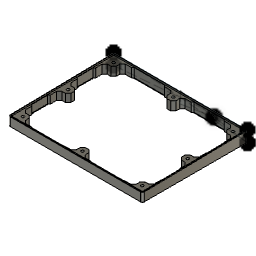
case (Autodesk Fusion 360 design; units mm, degrees)
Autodesk Fusion 360 part; units mm, degrees
sketch "Sketch1" plane through (0, 0, 0) normal (0, 0, 1) x (1, 0, 0)
  line L0 (0, 0) -> (294.692, 0)
  line L1 (294.692, 0) -> (294.692, 230.4)
  line L2 (294.692, 230.4) -> (0, 230.4)
  line L3 (0, 230.4) -> (0, 0)
  line L4 (-2, 232.4) -> (296.692, 232.4)
  line L5 (296.692, 232.4) -> (296.692, -2)
  line L6 (296.692, -2) -> (-2, -2)
  line L7 (-2, -2) -> (-2, 232.4)
  line L8 (4, 226.4) -> (290.692, 226.4)
  line L9 (290.692, 226.4) -> (290.692, 4)
  line L10 (290.692, 4) -> (4, 4)
  line L11 (4, 4) -> (4, 226.4)
  line L12 (-2, 232.4) -> (296.692, -2) construction
  line L13 (-2, -2) -> (296.692, 232.4) construction
  line L14 (147.346, 232.4) -> (147.346, -2) construction
  line L15 (296.692, 115.2) -> (-2, 115.2) construction
  line L16 (4, 226.4) -> (24, 226.4)
  line L17 (24, 226.4) -> (24, 206.4)
  line L18 (24, 206.4) -> (4, 206.4)
  line L19 (4, 206.4) -> (4, 226.4)
  line L20 (137.346, 226.4) -> (157.346, 226.4)
  line L21 (157.346, 226.4) -> (157.346, 206.4)
  line L22 (157.346, 206.4) -> (137.346, 206.4)
  line L23 (137.346, 206.4) -> (137.346, 226.4)
  line L24 (290.692, 226.4) -> (270.692, 226.4)
  line L25 (270.692, 226.4) -> (270.692, 206.4)
  line L26 (270.692, 206.4) -> (290.692, 206.4)
  line L27 (290.692, 206.4) -> (290.692, 226.4)
  line L28 (4, 125.2) -> (24, 125.2)
  line L29 (24, 125.2) -> (24, 105.2)
  line L30 (24, 105.2) -> (4, 105.2)
  line L31 (4, 105.2) -> (4, 125.2)
  line L32 (290.692, 125.2) -> (270.692, 125.2)
  line L33 (270.692, 125.2) -> (270.692, 105.2)
  line L34 (270.692, 105.2) -> (290.692, 105.2)
  line L35 (290.692, 105.2) -> (290.692, 125.2)
  line L36 (4, 4) -> (24, 4)
  line L37 (24, 4) -> (24, 24)
  line L38 (24, 24) -> (4, 24)
  line L39 (4, 24) -> (4, 4)
  line L40 (137.346, 4) -> (157.346, 4)
  line L41 (157.346, 4) -> (157.346, 24)
  line L42 (157.346, 24) -> (137.346, 24)
  line L43 (137.346, 24) -> (137.346, 4)
  line L44 (290.692, 4) -> (270.692, 4)
  line L45 (270.692, 4) -> (270.692, 24)
  line L46 (270.692, 24) -> (290.692, 24)
  line L47 (290.692, 24) -> (290.692, 4)
  line L48 (4, 206.4) -> (24, 226.4) construction
  line L49 (4, 226.4) -> (24, 206.4) construction
  line L50 (137.346, 226.4) -> (157.346, 206.4) construction
  line L51 (137.346, 206.4) -> (157.346, 226.4) construction
  line L52 (270.692, 226.4) -> (290.692, 206.4) construction
  line L53 (270.692, 206.4) -> (290.692, 226.4) construction
  line L54 (290.692, 125.2) -> (270.692, 105.2) construction
  line L55 (270.692, 125.2) -> (290.692, 105.2) construction
  line L56 (270.692, 4) -> (290.692, 24) construction
  line L57 (270.692, 24) -> (290.692, 4) construction
  line L58 (137.346, 4) -> (157.346, 24) construction
  line L59 (137.346, 24) -> (157.346, 4) construction
  line L60 (24, 24) -> (4, 4) construction
  line L61 (4, 24) -> (24, 4) construction
  line L62 (4, 125.2) -> (24, 105.2) construction
  line L63 (4, 105.2) -> (24, 125.2) construction
  circle A0 centre (14, 216.4) radius 3
  circle A1 centre (147.346, 216.4) radius 3
  circle A2 centre (14, 115.2) radius 3
  circle A3 centre (14, 14) radius 3
  circle A4 centre (147.346, 14) radius 3
  circle A5 centre (280.692, 14) radius 3
  circle A6 centre (280.692, 115.2) radius 3
  circle A7 centre (280.692, 216.4) radius 3
  line L64 (44, 226.4) -> (44, 230.4)
  line L65 (117.346, 230.4) -> (177.346, 230.4)
  line L66 (177.346, 230.4) -> (177.346, 226.4)
  line L67 (177.346, 226.4) -> (117.346, 226.4)
  line L68 (117.346, 226.4) -> (117.346, 230.4)
  line L69 (250.692, 226.4) -> (250.692, 230.4)
  line L70 (290.692, 186.4) -> (294.692, 186.4)
  line L71 (4, 186.4) -> (0, 186.4)
  line L72 (0, 145.2) -> (4, 145.2)
  line L73 (4, 145.2) -> (4, 85.2)
  line L74 (4, 85.2) -> (0, 85.2)
  line L75 (0, 85.2) -> (0, 145.2)
  line L76 (294.692, 145.2) -> (290.692, 145.2)
  line L77 (290.692, 145.2) -> (290.692, 85.2)
  line L78 (290.692, 85.2) -> (294.692, 85.2)
  line L79 (294.692, 85.2) -> (294.692, 145.2)
  line L80 (4, 44) -> (0, 44)
  line L81 (44, 4) -> (44, 0)
  line L82 (117.346, 4) -> (177.346, 4)
  line L83 (177.346, 4) -> (177.346, 0)
  line L84 (177.346, 0) -> (117.346, 0)
  line L85 (117.346, 0) -> (117.346, 4)
  line L86 (250.692, 4) -> (250.692, 0)
  line L87 (290.692, 44) -> (294.692, 44)
  line L88 (250.692, 1) -> (177.346, 1)
  line L89 (250.692, 4) -> (246.692, 0)
  line L90 (177.346, 4) -> (181.346, 0)
  line L91 (293.692, 44) -> (293.692, 85.2)
  line L92 (290.692, 44) -> (294.692, 48)
  line L93 (290.692, 85.2) -> (294.692, 81.2)
  line L94 (250.692, 229.4) -> (177.346, 229.4)
  line L95 (250.692, 226.4) -> (246.692, 230.4)
  line L96 (177.346, 226.4) -> (181.346, 230.4)
  line L97 (117.346, 1) -> (44, 1)
  line L98 (117.346, 4) -> (113.346, 0)
  line L99 (44, 4) -> (48, 0)
  line L100 (1, 44) -> (1, 85.2)
  line L101 (4, 44) -> (0, 48)
  line L102 (4, 85.2) -> (0, 81.2)
  line L103 (1, 186.4) -> (1, 145.2)
  line L104 (4, 186.4) -> (0, 182.4)
  line L105 (4, 145.2) -> (0, 149.2)
  line L106 (117.346, 229.4) -> (44, 229.4)
  line L107 (117.346, 226.4) -> (113.346, 230.4)
  line L108 (44, 226.4) -> (48, 230.4)
  line L109 (293.692, 145.2) -> (293.692, 186.4)
  line L110 (290.692, 145.2) -> (294.692, 149.2)
  line L111 (290.692, 186.4) -> (294.692, 182.4)
  dimension "d1" = 294.692
  dimension "d2" = 230.4
  dimension "d3" = 2
  dimension "d4" = 2
  dimension "d5" = 2
  dimension "d6" = 2
  dimension "d7" = 4
  dimension "d8" = 4
  dimension "d9" = 4
  dimension "d10" = 4
  dimension "d11" = 20
  dimension "d12" = 20
  dimension "d13" = 20
  dimension "d14" = 20
  dimension "d15" = 20
  dimension "d16" = 20
  dimension "d17" = 20
  dimension "d18" = 20
  dimension "d19" = 20
  dimension "d20" = 20
  dimension "d21" = 20
  dimension "d22" = 20
  dimension "d23" = 20
  dimension "d24" = 20
  dimension "d25" = 20
  dimension "d26" = 20
  dimension "d27" = 6
  dimension "d28" = 6
  dimension "d29" = 6
  dimension "d30" = 6
  dimension "d31" = 6
  dimension "d32" = 6
  dimension "d33" = 6
  dimension "d34" = 6
  dimension "d35" = 20
  dimension "d36" = 20
  dimension "d37" = 20
  dimension "d38" = 20
  dimension "d39" = 20
  dimension "d40" = 20
  dimension "d41" = 20
  dimension "d42" = 20
  dimension "d43" = 20
  dimension "d44" = 20
  dimension "d45" = 20
  dimension "d46" = 20
  dimension "d47" = 20
  dimension "d48" = 20
  dimension "d49" = 20
  dimension "d50" = 20
  dimension "d51" = 1
  dimension "d52" = 4
  dimension "d53" = 4
  dimension "d54" = 1
  dimension "d55" = 4
  dimension "d56" = 4
  dimension "d57" = 1
  dimension "d58" = 4
  dimension "d59" = 4
  dimension "d60" = 1
  dimension "d61" = 4
  dimension "d62" = 4
  dimension "d63" = 1
  dimension "d64" = 4
  dimension "d65" = 4
  dimension "d66" = 1
  dimension "d67" = 4
  dimension "d68" = 4
  dimension "d69" = 1
  dimension "d70" = 4
  dimension "d71" = 4
  dimension "d72" = 1
  dimension "d73" = 4
  dimension "d74" = 4
  constraint horizontal L0
  constraint vertical L1
  constraint horizontal L2
  constraint vertical L3
  constraint coincident L0.start L3.end
  constraint horizontal L4
  constraint vertical L5
  constraint horizontal L6
  constraint vertical L7
  constraint horizontal L8
  constraint vertical L9
  constraint horizontal L10
  constraint vertical L11
  constraint midpoint L4 L14.start
  constraint midpoint L6 L14.end
  constraint midpoint L5 L15.start
  constraint midpoint L7 L15.end
  constraint horizontal L16
  constraint vertical L17
  constraint horizontal L18
  constraint vertical L19
  constraint horizontal L20
  constraint vertical L21
  constraint horizontal L22
  constraint vertical L23
  constraint coincident L8 L20.start
  constraint horizontal L24
  constraint vertical L25
  constraint horizontal L26
  constraint vertical L27
  constraint horizontal L28
  constraint vertical L29
  constraint horizontal L30
  constraint vertical L31
  constraint coincident L11 L28.start
  constraint horizontal L32
  constraint vertical L33
  constraint horizontal L34
  constraint vertical L35
  constraint coincident L9 L32.start
  constraint horizontal L36
  constraint vertical L37
  constraint horizontal L38
  constraint vertical L39
  constraint horizontal L40
  constraint vertical L41
  constraint horizontal L42
  constraint vertical L43
  constraint coincident L10 L40.start
  constraint horizontal L44
  constraint vertical L45
  constraint horizontal L46
  constraint vertical L47
  constraint symmetric L14 L21 L23
  constraint symmetric L15 L28 L30
  constraint symmetric L15 L32 L34
  constraint symmetric L14 L41 L43
  constraint midpoint L48 A0.centre
  constraint midpoint L50 A1.centre
  constraint midpoint L63 A2.centre
  constraint midpoint L61 A3.centre
  constraint midpoint L59 A4.centre
  constraint midpoint L57 A5.centre
  constraint midpoint L55 A6.centre
  constraint midpoint L52 A7.centre
  constraint coincident L8 L64.start
  constraint coincident L2 L64.end
  constraint perpendicular L2 L64
  constraint horizontal L65
  constraint vertical L66
  constraint horizontal L67
  constraint vertical L68
  constraint coincident L8 L66.end
  constraint coincident L2 L65.start
  constraint coincident L8 L69.start
  constraint coincident L2 L69.end
  constraint perpendicular L2 L69
  constraint coincident L9 L70.start
  constraint coincident L1 L70.end
  constraint perpendicular L1 L70
  constraint coincident L11 L71.start
  constraint coincident L3 L71.end
  constraint perpendicular L3 L71
  constraint horizontal L72
  constraint vertical L73
  constraint horizontal L74
  constraint vertical L75
  constraint coincident L11 L73.end
  constraint coincident L3 L72.start
  constraint horizontal L76
  constraint vertical L77
  constraint horizontal L78
  constraint vertical L79
  constraint coincident L9 L77.end
  constraint coincident L1 L76.start
  constraint coincident L11 L80.start
  constraint coincident L3 L80.end
  constraint perpendicular L3 L80
  constraint coincident L10 L81.start
  constraint coincident L0 L81.end
  constraint perpendicular L0 L81
  constraint horizontal L82
  constraint vertical L83
  constraint horizontal L84
  constraint vertical L85
  constraint coincident L0 L83.end
  constraint coincident L10 L82.start
  constraint coincident L10 L86.start
  constraint coincident L0 L86.end
  constraint perpendicular L0 L86
  constraint coincident L9 L87.start
  constraint coincident L1 L87.end
  constraint perpendicular L1 L87
  constraint coincident L86 L88.start
  constraint coincident L83 L88.end
  constraint perpendicular L83 L88
  constraint coincident L0 L89.end
  constraint coincident L0 L90.end
  constraint coincident L87 L91.start
  constraint coincident L78 L91.end
  constraint perpendicular L78 L91
  constraint coincident L1 L92.end
  constraint coincident L1 L93.end
  constraint coincident L69 L94.start
  constraint coincident L66 L94.end
  constraint perpendicular L66 L94
  constraint coincident L2 L95.end
  constraint coincident L2 L96.end
  constraint coincident L85 L97.start
  constraint coincident L81 L97.end
  constraint perpendicular L81 L97
  constraint coincident L0 L98.end
  constraint coincident L0 L99.end
  constraint coincident L80 L100.start
  constraint coincident L74 L100.end
  constraint perpendicular L74 L100
  constraint coincident L3 L101.end
  constraint coincident L3 L102.end
  constraint coincident L71 L103.start
  constraint coincident L72 L103.end
  constraint perpendicular L72 L103
  constraint coincident L3 L104.end
  constraint coincident L3 L105.end
  constraint coincident L68 L106.start
  constraint coincident L64 L106.end
  constraint perpendicular L64 L106
  constraint coincident L2 L107.end
  constraint coincident L2 L108.end
  constraint coincident L76 L109.start
  constraint coincident L70 L109.end
  constraint perpendicular L70 L109
  constraint coincident L1 L110.end
  constraint coincident L1 L111.end
  measures "d1" distance of L0.start L0.end
  measures "d2" distance of L0.start L2.end
  measures "d3" distance of L3 L7
  measures "d4" distance of L2 L4
  measures "d5" distance of L1 L5
  measures "d6" distance of L0 L6
  measures "d7" distance of L2 L8
  measures "d8" distance of L3 L11
  measures "d9" distance of L1 L9
  measures "d10" distance of L0 L10
  measures "d11" distance of L8.start L16.end
  measures "d12" distance of L8.start L18.end
  measures "d13" distance of L20.start L20.end
  measures "d14" distance of L20.start L22.end
  measures "d15" distance of L8.end L24.end
  measures "d16" distance of L8.end L26.end
  measures "d17" distance of L28.start L28.end
  measures "d18" distance of L28.start L30.end
  measures "d19" distance of L32.start L32.end
  measures "d20" distance of L32.start L34.end
  measures "d21" distance of L10.end L36.end
  measures "d22" distance of L10.end L38.end
  measures "d23" distance of L40.start L40.end
  measures "d24" distance of L40.start L42.end
  measures "d25" distance of L9.end L44.end
  measures "d26" distance of L9.end L46.end
  measures "d27" diameter of A0
  measures "d28" diameter of A1
  measures "d29" diameter of A2
  measures "d30" diameter of A3
  measures "d31" diameter of A4
  measures "d32" diameter of A5
  measures "d33" diameter of A6
  measures "d34" diameter of A7
  measures "d35" distance of L16.end L64.start
  measures "d36" distance of L20.start L67.end
  measures "d37" distance of L20.end L66.end
  measures "d38" distance of L24.end L69.start
  measures "d39" distance of L26.end L70.start
  measures "d40" distance of L18.end L71.start
  measures "d41" distance of L28.start L72.end
  measures "d42" distance of L30.end L73.end
  measures "d43" distance of L32.start L76.end
  measures "d44" distance of L34.end L77.end
  measures "d45" distance of L38.end L80.start
  measures "d46" distance of L36.end L81.start
  measures "d47" distance of L40.start L82.start
  measures "d48" distance of L40.end L82.end
  measures "d49" distance of L44.end L86.start
  measures "d50" distance of L46.end L87.start
  measures "d51" distance of L0 L88
  measures "d52" distance of L86.end L89.end
  measures "d53" distance of L83.end L90.end
  measures "d54" distance of L1 L91
  measures "d55" distance of L87.end L92.end
  measures "d56" distance of L78.end L93.end
  measures "d57" distance of L2 L94
  measures "d58" distance of L69.end L95.end
  measures "d59" distance of L65.end L96.end
  measures "d60" distance of L0 L97
  measures "d61" distance of L84.end L98.end
  measures "d62" distance of L81.end L99.end
  measures "d63" distance of L3 L100
  measures "d64" distance of L80.end L101.end
  measures "d65" distance of L74.end L102.end
  measures "d66" distance of L3 L103
  measures "d67" distance of L71.end L104.end
  measures "d68" distance of L72.start L105.end
  measures "d69" distance of L2 L106
  measures "d70" distance of L65.start L107.end
  measures "d71" distance of L64.end L108.end
  measures "d72" distance of L1 L109
  measures "d73" distance of L76.start L110.end
  measures "d74" distance of L70.end L111.end
extrude "Extrude1" add sketch "Sketch1" along normal blind 20 contours L0 L3 L10 L11 L36 L39 L80 L81 | L0 L81 L97 L99 | L3 L80 L100 L101 | L0 L97 L98 L99 | L81 L97 L99 | L3 L100 L101 L102 | L80 L100 L101 | L0 L85 L97 L98 | L3 L74 L100 L102 | L0 L10 L40 L82 L83 L84 L85 | L85 L97 L98 | L10 L11 L36 L37 L38 L39 | L3 L11 L31 L72 L73 L74 L75 | L74 L100 L102 | L0 L83 L88 L90 | L10 L40 L41 L42 L43 L82 | L3 L72 L103 L105 | L11 L28 L29 L30 L31 L73 | L0 L88 L89 L90 | L83 L88 L90 | L3 L103 L104 L105 | L72 L103 L105 | L0 L86 L88 L89 | L3 L71 L103 L104 | L0 L1 L9 L10 L44 L47 L86 L87 | L86 L88 L89 | L2 L3 L8 L11 L16 L19 L64 L71 | L71 L103 L104 | L9 L10 L44 L45 L46 L47 | L8 L11 L16 L17 L18 L19 | L1 L87 L91 L92 | L2 L64 L106 L108 | L1 L91 L92 L93 | L87 L91 L92 | L2 L106 L107 L108 | L64 L106 L108 | L1 L78 L91 L93 | L2 L68 L106 L107 | L1 L9 L35 L76 L77 L78 L79 | L78 L91 L93 | L2 L8 L20 L65 L66 L67 L68 | L68 L106 L107 | L1 L76 L109 L110 | L9 L32 L33 L34 L35 L77 | L2 L66 L94 L96 | L8 L20 L21 L22 L23 L67 | L1 L109 L110 L111 | L76 L109 L110 | L2 L94 L95 L96 | L66 L94 L96 | L1 L70 L109 L111 | L2 L69 L94 L95 | L1 L2 L8 L9 L24 L27 L69 L70 | L70 L109 L111 | L69 L94 L95 | L8 L9 L24 L25 L26 L27 | L4 L5 L6 L7
chamfer "Chamfer1" distance 6 angle 45 28 edges at (270.692, 4, 10) (270.692, 24, 10) (290.692, 24, 10) (290.692, 105.2, 10) (270.692, 105.2, 10) (270.692, 125.2, 10) (290.692, 125.2, 10) (157.346, 4, 10) (157.346, 24, 10) (137.346, 4, 10) (137.346, 24, 10) (290.692, 206.4, 10) (270.692, 206.4, 10) (270.692, 226.4, 10) (157.346, 206.4, 10) (157.346, 226.4, 10) (137.346, 206.4, 10) (137.346, 226.4, 10) (24, 206.4, 10) (24, 226.4, 10) (4, 206.4, 10) (4, 125.2, 10) (24, 125.2, 10) (24, 105.2, 10) (4, 105.2, 10) (4, 24, 10) (24, 24, 10) (24, 4, 10)
sketch "Sketch2" plane through (0, 0, 20) normal (0, 0, 1) x (-1, 0, 0)
  line L0 (-24, -18) -> (-18, -24)
  line L1 (-18, -24) -> (-10, -24)
  line L2 (-10, -24) -> (-4, -30)
  line L3 (-4, -30) -> (-4, -44)
  line L4 (-4, -44) -> (-1, -47)
  line L5 (-1, -47) -> (-1, -82.2)
  line L6 (-1, -82.2) -> (-4, -85.2)
  line L7 (-4, -85.2) -> (-4, -99.2)
  line L8 (-4, -99.2) -> (-10, -105.2)
  line L9 (-10, -105.2) -> (-18, -105.2)
  line L10 (-18, -105.2) -> (-24, -111.2)
  line L11 (-24, -111.2) -> (-24, -119.2)
  line L12 (-24, -119.2) -> (-18, -125.2)
  line L13 (-18, -125.2) -> (-10, -125.2)
  line L14 (-10, -125.2) -> (-4, -131.2)
  line L15 (-4, -131.2) -> (-4, -145.2)
  line L16 (-4, -145.2) -> (-1, -148.2)
  line L17 (-1, -148.2) -> (-1, -183.4)
  line L18 (-1, -183.4) -> (-4, -186.4)
  line L19 (-4, -186.4) -> (-4, -200.4)
  line L20 (-4, -200.4) -> (-10, -206.4)
  line L21 (-10, -206.4) -> (-18, -206.4)
  line L22 (-18, -206.4) -> (-24, -212.4)
  line L23 (-24, -212.4) -> (-24, -220.4)
  line L24 (-24, -220.4) -> (-30, -226.4)
  line L25 (-30, -226.4) -> (-44, -226.4)
  line L26 (-44, -226.4) -> (-47, -229.4)
  line L27 (-47, -229.4) -> (-114.346, -229.4)
  line L28 (-114.346, -229.4) -> (-117.346, -226.4)
  line L29 (-117.346, -226.4) -> (-131.346, -226.4)
  line L30 (-131.346, -226.4) -> (-137.346, -220.4)
  line L31 (-137.346, -220.4) -> (-137.346, -212.4)
  line L32 (-137.346, -212.4) -> (-143.346, -206.4)
  line L33 (-143.346, -206.4) -> (-151.346, -206.4)
  line L34 (-151.346, -206.4) -> (-157.346, -212.4)
  line L35 (-157.346, -212.4) -> (-157.346, -220.4)
  line L36 (-157.346, -220.4) -> (-163.346, -226.4)
  line L37 (-163.346, -226.4) -> (-177.346, -226.4)
  line L38 (-177.346, -226.4) -> (-180.346, -229.4)
  line L39 (-180.346, -229.4) -> (-247.692, -229.4)
  line L40 (-247.692, -229.4) -> (-250.692, -226.4)
  line L41 (-250.692, -226.4) -> (-264.692, -226.4)
  line L42 (-264.692, -226.4) -> (-270.692, -220.4)
  line L43 (-270.692, -220.4) -> (-270.692, -212.4)
  line L44 (-270.692, -212.4) -> (-276.692, -206.4)
  line L45 (-276.692, -206.4) -> (-284.692, -206.4)
  line L46 (-284.692, -206.4) -> (-290.692, -200.4)
  line L47 (-290.692, -200.4) -> (-290.692, -186.4)
  line L48 (-290.692, -186.4) -> (-293.692, -183.4)
  line L49 (-293.692, -183.4) -> (-293.692, -148.2)
  line L50 (-293.692, -148.2) -> (-290.692, -145.2)
  line L51 (-290.692, -145.2) -> (-290.692, -131.2)
  line L52 (-290.692, -131.2) -> (-284.692, -125.2)
  line L53 (-284.692, -125.2) -> (-276.692, -125.2)
  line L54 (-276.692, -125.2) -> (-270.692, -119.2)
  line L55 (-270.692, -119.2) -> (-270.692, -111.2)
  line L56 (-270.692, -111.2) -> (-276.692, -105.2)
  line L57 (-276.692, -105.2) -> (-284.692, -105.2)
  line L58 (-284.692, -105.2) -> (-290.692, -99.2)
  line L59 (-290.692, -99.2) -> (-290.692, -85.2)
  line L60 (-290.692, -85.2) -> (-293.692, -82.2)
  line L61 (-293.692, -82.2) -> (-293.692, -47)
  line L62 (-293.692, -47) -> (-290.692, -44)
  line L63 (-290.692, -44) -> (-290.692, -30)
  line L64 (-290.692, -30) -> (-284.692, -24)
  line L65 (-284.692, -24) -> (-276.692, -24)
  line L66 (-276.692, -24) -> (-270.692, -18)
  line L67 (-270.692, -18) -> (-270.692, -10)
  line L68 (-270.692, -10) -> (-264.692, -4)
  line L69 (-264.692, -4) -> (-250.692, -4)
  line L70 (-250.692, -4) -> (-247.692, -1)
  line L71 (-247.692, -1) -> (-180.346, -1)
  line L72 (-180.346, -1) -> (-177.346, -4)
  line L73 (-177.346, -4) -> (-163.346, -4)
  line L74 (-163.346, -4) -> (-157.346, -10)
  line L75 (-157.346, -10) -> (-157.346, -18)
  line L76 (-157.346, -18) -> (-151.346, -24)
  line L77 (-151.346, -24) -> (-143.346, -24)
  line L78 (-143.346, -24) -> (-137.346, -18)
  line L79 (-137.346, -18) -> (-137.346, -10)
  line L80 (-137.346, -10) -> (-131.346, -4)
  line L81 (-131.346, -4) -> (-117.346, -4)
  line L82 (-117.346, -4) -> (-114.346, -1)
  line L83 (-114.346, -1) -> (-47, -1)
  line L84 (-47, -1) -> (-44, -4)
  line L85 (-44, -4) -> (-30, -4)
  line L86 (-30, -4) -> (-24, -10)
  line L87 (-24, -10) -> (-24, -18)
  circle A0 centre (-280.692, -115.2) radius 3
  circle A1 centre (-280.692, -216.4) radius 3
  circle A2 centre (-14, -115.2) radius 3
  circle A3 centre (-14, -216.4) radius 3
  circle A4 centre (-147.346, -216.4) radius 3
  circle A5 centre (-147.346, -14) radius 3
  circle A6 centre (-280.692, -14) radius 3
  circle A7 centre (-14, -14) radius 3
  line L88 (2, 2) -> (-296.692, 2)
  line L89 (-296.692, 2) -> (-296.692, -232.4)
  line L90 (-296.692, -232.4) -> (2, -232.4)
  line L91 (2, -232.4) -> (2, 2)
  line L92 (-294.692, 0) -> (0, 0)
  line L93 (0, 0) -> (0, -230.4)
  line L94 (0, -230.4) -> (-294.692, -230.4)
  line L95 (-294.692, -230.4) -> (-294.692, 0)
  dimension "d78" = 2
  dimension "d79" = 2
  dimension "d80" = 2
  dimension "d81" = 2
  constraint horizontal L92
  constraint vertical L93
  constraint horizontal L94
  constraint vertical L95
  measures "d78" distance of L88 L92
  measures "d79" distance of L89 L95
  measures "d80" distance of L90 L94
  measures "d81" distance of L91 L93
sketch "Sketch3" plane through (-2, 0, 0) normal (-1, 0, 0) x (0, -1, 0)
  line L0 (-232.4, 0) -> (2, 0)
  line L1 (2, 0) -> (2, 20)
  line L2 (2, 20) -> (-232.4, 20)
  line L3 (-232.4, 20) -> (-232.4, 0)
  line L4 (2, 0) -> (2, 16)
  line L5 (2, 16) -> (-232.4, 20)
  dimension "d82" = 16
  constraint coincident L0.end L1.start
  constraint perpendicular L0 L4
  constraint coincident L2.end L3.start
  measures "d82" distance of L0.end L4.end
extrude "Extrude2" cut sketch "Sketch3" against normal through all contours L1 L2 L5
extrude "Extrude3" add sketch "Sketch2" against normal through all contours L88 L89 L90 L91
extrude "Extrude4" add 1 faces at (196.4613, -1.3333, 20) along direction (0, 0, 1) blind 3
extrude "Extrude5" add sketch "Sketch1" against normal blind 2 contours L4 L5 L6 L7
sketch "Sketch4" plane through (-2, 0, 0) normal (-1, 0, 0) x (0, -1, 0)
  line L0 (-232.4, 23) -> (-232.4, -2)
  line L1 (-232.4, -2) -> (2, -2)
  line L2 (2, -2) -> (2, 23)
  line L3 (2, 23) -> (-232.4, 23)
  line L4 (2, -2) -> (2, 19)
  line L5 (2, 19) -> (-232.4, 23)
  dimension "d89" = 21
  constraint coincident L1.end L2.start
  constraint perpendicular L1 L4
  constraint coincident L0.start L3.end
  measures "d89" distance of L1.end L4.end
extrude "Extrude6" cut sketch "Sketch4" against normal through all contours L2 L3 L5
sketch "Sketch5" plane through (0, 232.4, 0) normal (0, 1, 0) x (-1, 0, 0)
  line L0 (2, -2) -> (2, 23)
  line L1 (2, 23) -> (-296.692, 23)
  line L2 (-296.692, 23) -> (-296.692, -2)
  line L3 (-296.692, -2) -> (2, -2)
  line L4 (-296.692, -2) -> (2, 23) construction
  line L5 (2, -2) -> (-296.692, 23) construction
  line L6 (-147.346, 23) -> (-147.346, -2) construction
  line L7 (-296.692, -2) -> (-147.346, 23) construction
  line L8 (-147.346, -2) -> (-296.692, 23) construction
  circle A0 centre (-222.019, 10.5) radius 5.6
  circle A1 centre (-222.019, 10.5) radius 6.8
  line L9 (-224.0975, 15.7) -> (-219.9405, 15.7)
  line L10 (-224.0975, 5.3) -> (-219.9405, 5.3)
  dimension "d91" = 11.2
  dimension "d92" = 13.6
  dimension "d103" = 10.4
  constraint coincident L2.end L3.start
  constraint coincident L0.end L1.start
  constraint coincident L0.start L3.end
  constraint coincident L1.end L2.start
  constraint midpoint L1 L6.start
  constraint midpoint L3 L6.end
  constraint midpoint L8 A0.centre
  constraint concentric A0 A1
  constraint coincident A0 L9.start
  constraint coincident A0 L9.end
  constraint horizontal L9
  constraint coincident A0 L10.start
  constraint coincident A0 L10.end
  constraint parallel L9 L10
  constraint equal L9 L10
  measures "d91" diameter of A0
  measures "d92" diameter of A1
  measures "d103" distance of L9 L10
extrude "Extrude7" cut sketch "Sketch5" against normal blind 3 contours A0 L9 L10 | A0 L9 | A0 L10 | A1
extrude "Extrude8" add sketch "Sketch5" against normal blind 3 contours A1
fillet "Fillet1" radius 2 8 edges at (294.692, 0, 17.5341) (294.692, 230.4, 21.4659) (0, 0, 17.5341) (0, 230.4, 21.4659) (0, 230.4, -1) (294.692, 230.4, -1) (294.692, 0, -1) (0, 0, -1)
fillet "Fillet2" radius 4 4 edges at (296.692, -2, 8.5) (296.692, 232.4, 10.5) (-2, 232.4, 10.5) (-2, -2, 8.5)
fillet "Fillet3" radius 1 16 edges at (295.5204, 231.2284, -2) (296.692, 115.2, -2) (295.5204, -0.8284, -2) (147.346, -2, -2) (-0.8284, -0.8284, -2) (-2, 115.2, -2) (-0.8284, 231.2284, -2) (147.346, 232.4, -2) (-0.8284, 231.2284, 22.98) (-2, 115.2, 21) (-0.8284, -0.8284, 19.02) (147.346, -2, 19) (295.5204, -0.8284, 19.02) (296.692, 115.2, 21) (295.5204, 231.2284, 22.98) (147.346, 232.4, 23)
extrude "Extrude9" add sketch "Sketch5" against normal blind 3 contours A0 L9 | A0 L10
equation "d89 = 16 mm + 2 mm + 3 mm"
